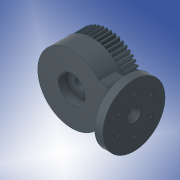
# Autodesk Inventor part: BA013
Saved by Autodesk Inventor 2017 SP1 (Build 210196100, 196)
## iProperties
Created: 2017-06-27
Part Number: BA013
Material: ABS Plastic
Document SubType Name: Modeling
Designer: zallen
Density: 1.06 g/cm^3
Appearance: CR Dark Blue
Author: zallen
Autodesk Inventor part; units mm, degrees
ref_plane "YZ Plane" through (0, 0, 0) normal (1, 0, 0) x (0, 1, 0)
ref_plane "XZ Plane" through (0, 0, 0) normal (0, 1, 0) x (-1, 0, 0)
ref_plane "XY Plane" through (0, 0, 0) normal (0, 0, 1) x (1, 0, 0)
sketch "Sketch1" plane through (0, 0, 0) normal (0, 0, 1) x (1, 0, 0)
  circle A0 centre (0, 0) radius 36.25
  circle A1 centre (0, 0) radius 7.5
  line L0 (0, 0) -> (67.2646, 0) construction
  arc A2 (40.2053, 0.75) -> (36.2053, 1.8) centre (34.4332, -13.095) ccw
  arc A3 (36.2053, -1.8) -> (40.2053, -0.75) centre (34.4332, 13.095) ccw
  arc A4 (40.2053, -0.75) -> (40.2053, 0.75) centre (20.2194, 0) ccw
  arc A5 (36.2053, -1.8) -> (36.2053, 1.8) centre (0, 0) ccw
  arc A6 (39.9823, 4.295) -> (39.7943, 5.7831) centre (20.0599, 2.5342) ccw
  arc A7 (39.7943, 5.7831) -> (35.6942, 6.3235) centre (35.8029, -8.6761) ccw
  arc A8 (36.1454, 2.7519) -> (39.9823, 4.295) centre (32.5204, 17.3073) ccw
  circle A9 centre (0, 0) radius 36.25
  arc A10 (39.1287, 9.2722) -> (38.7556, 10.7251) centre (19.5841, 5.0283) ccw
  arc A11 (38.7556, 10.7251) -> (34.6202, 10.7473) centre (36.608, -4.1204) ccw
  arc A12 (35.5155, 7.2604) -> (39.1287, 9.2722) centre (30.0948, 21.2467) ccw
  circle A13 centre (0, 0) radius 36.25
  arc A14 (37.658, 14.1032) -> (37.1058, 15.4979) centre (18.7995, 7.4432) ccw
  arc A15 (37.1058, 15.4979) -> (33.0002, 15.0017) centre (36.8357, 0.5003) ccw
  arc A16 (34.3254, 11.6545) -> (37.658, 14.1032) centre (27.1946, 24.8511) ccw
  circle A17 centre (0, 0) radius 36.25
  arc A18 (35.5935, 18.7118) -> (34.8708, 20.0263) centre (17.7184, 9.7407) ccw
  arc A19 (34.8708, 20.0263) -> (30.8598, 19.0194) centre (36.4826, 5.1131) ccw
  arc A20 (32.5941, 15.8647) -> (35.5935, 18.7118) centre (23.8655, 28.0635) ccw
  circle A21 centre (0, 0) radius 36.25
  arc A22 (32.9676, 23.0253) -> (32.0859, 24.2388) centre (16.3578, 11.8846) ccw
  arc A23 (32.0859, 24.2388) -> (28.2327, 22.7372) centre (35.554, 9.6453) ccw
  arc A24 (30.3487, 19.8247) -> (32.9676, 23.0253) centre (20.16, 30.8333) ccw
  circle A25 centre (0, 0) radius 36.25
  arc A26 (29.8218, 26.9757) -> (28.795, 28.0691) centre (14.7393, 13.8411) ccw
  arc A27 (28.795, 28.0691) -> (25.1603, 26.0964) centre (34.0648, 14.0253) ccw
  arc A28 (27.6247, 23.4721) -> (29.8218, 26.9757) centre (16.1366, 33.1169) ccw
  circle A29 centre (0, 0) radius 36.25
  arc A30 (26.2057, 30.5006) -> (25.0499, 31.4568) centre (12.8883, 15.5793) ccw
  arc A31 (25.0499, 31.4568) -> (21.6912, 29.044) centre (32.0384, 18.1842) ccw
  arc A32 (24.465, 26.7493) -> (26.2057, 30.5006) centre (11.8587, 34.8783) ccw
  circle A33 centre (0, 0) radius 36.25
  arc A34 (22.1763, 33.5446) -> (20.9098, 34.3483) centre (10.8341, 17.0718) ccw
  arc A35 (20.9098, 34.3483) -> (17.88, 31.5336) centre (29.5066, 22.0563) ccw
  arc A36 (20.9196, 29.6046) -> (22.1763, 33.5446) centre (7.3938, 36.0895) ccw
  circle A37 centre (0, 0) radius 36.25
  arc A38 (17.7972, 36.0595) -> (16.44, 36.6982) centre (8.609, 18.295) ccw
  arc A39 (16.44, 36.6982) -> (13.7868, 33.5259) centre (26.5096, 25.5805) ccw
  arc A40 (17.0441, 31.9931) -> (17.7972, 36.0595) centre (2.8123, 36.7316) ccw
  circle A41 centre (0, 0) radius 36.25
  arc A42 (13.1374, 38.0057) -> (11.7108, 38.4693) centre (6.2481, 19.2297) ccw
  arc A43 (11.7108, 38.4693) -> (9.4761, 34.9895) centre (23.0945, 28.7013) ccw
  arc A44 (12.8999, 33.877) -> (13.1374, 38.0057) centre (-1.8136, 36.7945) ccw
  circle A45 centre (0, 0) radius 36.25
  arc A46 (8.2704, 39.3526) -> (6.797, 39.6337) centre (3.7887, 19.8612) ccw
  arc A47 (6.797, 39.6337) -> (5.0161, 35.9013) centre (19.3151, 31.3695) ccw
  arc A48 (8.5523, 35.2267) -> (8.2704, 39.3526) centre (-6.4109, 36.277) ccw
  circle A49 centre (0, 0) radius 36.25
  arc A50 (3.273, 40.0789) -> (1.776, 40.173) centre (1.2696, 20.1795) ccw
  arc A51 (1.776, 40.173) -> (0.4769, 36.2469) centre (15.2312, 33.543) ccw
  arc A52 (4.0698, 36.0208) -> (3.273, 40.0789) centre (-10.907, 35.1875) ccw
  circle A53 centre (0, 0) radius 36.25
  arc A54 (-1.776, 40.173) -> (-3.273, 40.0789) centre (-1.2696, 20.1795) ccw
  arc A55 (-3.273, 40.0789) -> (-4.0698, 36.0208) centre (10.907, 35.1875) ccw
  arc A56 (-0.4769, 36.2469) -> (-1.776, 40.173) centre (-15.2312, 33.543) ccw
  circle A57 centre (0, 0) radius 36.25
  arc A58 (-6.797, 39.6337) -> (-8.2704, 39.3526) centre (-3.7887, 19.8612) ccw
  arc A59 (-8.2704, 39.3526) -> (-8.5523, 35.2267) centre (6.4109, 36.277) ccw
  arc A60 (-5.0161, 35.9013) -> (-6.797, 39.6337) centre (-19.3151, 31.3695) ccw
  circle A61 centre (0, 0) radius 36.25
  arc A62 (-11.7108, 38.4693) -> (-13.1374, 38.0057) centre (-6.2481, 19.2297) ccw
  arc A63 (-13.1374, 38.0057) -> (-12.8999, 33.877) centre (1.8136, 36.7945) ccw
  arc A64 (-9.4761, 34.9895) -> (-11.7108, 38.4693) centre (-23.0945, 28.7013) ccw
  circle A65 centre (0, 0) radius 36.25
  arc A66 (-16.44, 36.6982) -> (-17.7972, 36.0595) centre (-8.609, 18.295) ccw
  arc A67 (-17.7972, 36.0595) -> (-17.0441, 31.9931) centre (-2.8123, 36.7316) ccw
  arc A68 (-13.7868, 33.5259) -> (-16.44, 36.6982) centre (-26.5096, 25.5805) ccw
  circle A69 centre (0, 0) radius 36.25
  arc A70 (-20.9098, 34.3483) -> (-22.1763, 33.5446) centre (-10.8341, 17.0718) ccw
  arc A71 (-22.1763, 33.5446) -> (-20.9196, 29.6046) centre (-7.3938, 36.0895) ccw
  arc A72 (-17.88, 31.5336) -> (-20.9098, 34.3483) centre (-29.5066, 22.0563) ccw
  circle A73 centre (0, 0) radius 36.25
  arc A74 (-25.0499, 31.4568) -> (-26.2057, 30.5006) centre (-12.8883, 15.5793) ccw
  arc A75 (-26.2057, 30.5006) -> (-24.465, 26.7493) centre (-11.8587, 34.8783) ccw
  arc A76 (-21.6912, 29.044) -> (-25.0499, 31.4568) centre (-32.0384, 18.1842) ccw
  circle A77 centre (0, 0) radius 36.25
  arc A78 (-28.795, 28.0691) -> (-29.8218, 26.9757) centre (-14.7393, 13.8411) ccw
  arc A79 (-29.8218, 26.9757) -> (-27.6247, 23.4721) centre (-16.1366, 33.1169) ccw
  arc A80 (-25.1603, 26.0964) -> (-28.795, 28.0691) centre (-34.0648, 14.0253) ccw
  circle A81 centre (0, 0) radius 36.25
  arc A82 (-32.0859, 24.2388) -> (-32.9676, 23.0253) centre (-16.3578, 11.8846) ccw
  arc A83 (-32.9676, 23.0253) -> (-30.3487, 19.8247) centre (-20.16, 30.8333) ccw
  arc A84 (-28.2327, 22.7372) -> (-32.0859, 24.2388) centre (-35.554, 9.6453) ccw
  circle A85 centre (0, 0) radius 36.25
  arc A86 (-34.8708, 20.0263) -> (-35.5935, 18.7118) centre (-17.7184, 9.7407) ccw
  arc A87 (-35.5935, 18.7118) -> (-32.5941, 15.8647) centre (-23.8655, 28.0635) ccw
  arc A88 (-30.8598, 19.0194) -> (-34.8708, 20.0263) centre (-36.4826, 5.1131) ccw
  circle A89 centre (0, 0) radius 36.25
  arc A90 (-37.1058, 15.4979) -> (-37.658, 14.1032) centre (-18.7995, 7.4432) ccw
  arc A91 (-37.658, 14.1032) -> (-34.3254, 11.6545) centre (-27.1946, 24.8511) ccw
  arc A92 (-33.0002, 15.0017) -> (-37.1058, 15.4979) centre (-36.8357, 0.5003) ccw
  circle A93 centre (0, 0) radius 36.25
  arc A94 (-38.7556, 10.7251) -> (-39.1287, 9.2722) centre (-19.5841, 5.0283) ccw
  arc A95 (-39.1287, 9.2722) -> (-35.5155, 7.2604) centre (-30.0948, 21.2467) ccw
  arc A96 (-34.6202, 10.7473) -> (-38.7556, 10.7251) centre (-36.608, -4.1204) ccw
  circle A97 centre (0, 0) radius 36.25
  arc A98 (-39.7943, 5.7831) -> (-39.9823, 4.295) centre (-20.0599, 2.5342) ccw
  arc A99 (-39.9823, 4.295) -> (-36.1454, 2.7519) centre (-32.5204, 17.3073) ccw
  arc A100 (-35.6942, 6.3235) -> (-39.7943, 5.7831) centre (-35.8029, -8.6761) ccw
  circle A101 centre (0, 0) radius 36.25
  arc A102 (-40.2053, 0.75) -> (-40.2053, -0.75) centre (-20.2194, 0) ccw
  arc A103 (-40.2053, -0.75) -> (-36.2053, -1.8) centre (-34.4332, 13.095) ccw
  arc A104 (-36.2053, 1.8) -> (-40.2053, 0.75) centre (-34.4332, -13.095) ccw
  circle A105 centre (0, 0) radius 36.25
  arc A106 (-39.9823, -4.295) -> (-39.7943, -5.7831) centre (-20.0599, -2.5342) ccw
  arc A107 (-39.7943, -5.7831) -> (-35.6942, -6.3235) centre (-35.8029, 8.6761) ccw
  arc A108 (-36.1454, -2.7519) -> (-39.9823, -4.295) centre (-32.5204, -17.3073) ccw
  circle A109 centre (0, 0) radius 36.25
  arc A110 (-39.1287, -9.2722) -> (-38.7556, -10.7251) centre (-19.5841, -5.0283) ccw
  arc A111 (-38.7556, -10.7251) -> (-34.6202, -10.7473) centre (-36.608, 4.1204) ccw
  arc A112 (-35.5155, -7.2604) -> (-39.1287, -9.2722) centre (-30.0948, -21.2467) ccw
  circle A113 centre (0, 0) radius 36.25
  arc A114 (-37.658, -14.1032) -> (-37.1058, -15.4979) centre (-18.7995, -7.4432) ccw
  arc A115 (-37.1058, -15.4979) -> (-33.0002, -15.0017) centre (-36.8357, -0.5003) ccw
  arc A116 (-34.3254, -11.6545) -> (-37.658, -14.1032) centre (-27.1946, -24.8511) ccw
  circle A117 centre (0, 0) radius 36.25
  arc A118 (-35.5935, -18.7118) -> (-34.8708, -20.0263) centre (-17.7184, -9.7407) ccw
  arc A119 (-34.8708, -20.0263) -> (-30.8598, -19.0194) centre (-36.4826, -5.1131) ccw
  arc A120 (-32.5941, -15.8647) -> (-35.5935, -18.7118) centre (-23.8655, -28.0635) ccw
  circle A121 centre (0, 0) radius 36.25
  arc A122 (-32.9676, -23.0253) -> (-32.0859, -24.2388) centre (-16.3578, -11.8846) ccw
  arc A123 (-32.0859, -24.2388) -> (-28.2327, -22.7372) centre (-35.554, -9.6453) ccw
  arc A124 (-30.3487, -19.8247) -> (-32.9676, -23.0253) centre (-20.16, -30.8333) ccw
  circle A125 centre (0, 0) radius 36.25
  arc A126 (-29.8218, -26.9757) -> (-28.795, -28.0691) centre (-14.7393, -13.8411) ccw
  arc A127 (-28.795, -28.0691) -> (-25.1603, -26.0964) centre (-34.0648, -14.0253) ccw
  arc A128 (-27.6247, -23.4721) -> (-29.8218, -26.9757) centre (-16.1366, -33.1169) ccw
  circle A129 centre (0, 0) radius 36.25
  arc A130 (-26.2057, -30.5006) -> (-25.0499, -31.4568) centre (-12.8883, -15.5793) ccw
  arc A131 (-25.0499, -31.4568) -> (-21.6912, -29.044) centre (-32.0384, -18.1842) ccw
  arc A132 (-24.465, -26.7493) -> (-26.2057, -30.5006) centre (-11.8587, -34.8783) ccw
  circle A133 centre (0, 0) radius 36.25
  arc A134 (-22.1763, -33.5446) -> (-20.9098, -34.3483) centre (-10.8341, -17.0718) ccw
  arc A135 (-20.9098, -34.3483) -> (-17.88, -31.5336) centre (-29.5066, -22.0563) ccw
  arc A136 (-20.9196, -29.6046) -> (-22.1763, -33.5446) centre (-7.3938, -36.0895) ccw
  circle A137 centre (0, 0) radius 36.25
  arc A138 (-17.7972, -36.0595) -> (-16.44, -36.6982) centre (-8.609, -18.295) ccw
  arc A139 (-16.44, -36.6982) -> (-13.7868, -33.5259) centre (-26.5096, -25.5805) ccw
  arc A140 (-17.0441, -31.9931) -> (-17.7972, -36.0595) centre (-2.8123, -36.7316) ccw
  circle A141 centre (0, 0) radius 36.25
  arc A142 (-13.1374, -38.0057) -> (-11.7108, -38.4693) centre (-6.2481, -19.2297) ccw
  arc A143 (-11.7108, -38.4693) -> (-9.4761, -34.9895) centre (-23.0945, -28.7013) ccw
  arc A144 (-12.8999, -33.877) -> (-13.1374, -38.0057) centre (1.8136, -36.7945) ccw
  circle A145 centre (0, 0) radius 36.25
  arc A146 (-8.2704, -39.3526) -> (-6.797, -39.6337) centre (-3.7887, -19.8612) ccw
  arc A147 (-6.797, -39.6337) -> (-5.0161, -35.9013) centre (-19.3151, -31.3695) ccw
  arc A148 (-8.5523, -35.2267) -> (-8.2704, -39.3526) centre (6.4109, -36.277) ccw
  circle A149 centre (0, 0) radius 36.25
  arc A150 (-3.273, -40.0789) -> (-1.776, -40.173) centre (-1.2696, -20.1795) ccw
  arc A151 (-1.776, -40.173) -> (-0.4769, -36.2469) centre (-15.2312, -33.543) ccw
  arc A152 (-4.0698, -36.0208) -> (-3.273, -40.0789) centre (10.907, -35.1875) ccw
  circle A153 centre (0, 0) radius 36.25
  arc A154 (1.776, -40.173) -> (3.273, -40.0789) centre (1.2696, -20.1795) ccw
  arc A155 (3.273, -40.0789) -> (4.0698, -36.0208) centre (-10.907, -35.1875) ccw
  arc A156 (0.4769, -36.2469) -> (1.776, -40.173) centre (15.2312, -33.543) ccw
  circle A157 centre (0, 0) radius 36.25
  arc A158 (6.797, -39.6337) -> (8.2704, -39.3526) centre (3.7887, -19.8612) ccw
  arc A159 (8.2704, -39.3526) -> (8.5523, -35.2267) centre (-6.4109, -36.277) ccw
  arc A160 (5.0161, -35.9013) -> (6.797, -39.6337) centre (19.3151, -31.3695) ccw
  circle A161 centre (0, 0) radius 36.25
  arc A162 (11.7108, -38.4693) -> (13.1374, -38.0057) centre (6.2481, -19.2297) ccw
  arc A163 (13.1374, -38.0057) -> (12.8999, -33.877) centre (-1.8136, -36.7945) ccw
  arc A164 (9.4761, -34.9895) -> (11.7108, -38.4693) centre (23.0945, -28.7013) ccw
  circle A165 centre (0, 0) radius 36.25
  arc A166 (16.44, -36.6982) -> (17.7972, -36.0595) centre (8.609, -18.295) ccw
  arc A167 (17.7972, -36.0595) -> (17.0441, -31.9931) centre (2.8123, -36.7316) ccw
  arc A168 (13.7868, -33.5259) -> (16.44, -36.6982) centre (26.5096, -25.5805) ccw
  circle A169 centre (0, 0) radius 36.25
  arc A170 (20.9098, -34.3483) -> (22.1763, -33.5446) centre (10.8341, -17.0718) ccw
  arc A171 (22.1763, -33.5446) -> (20.9196, -29.6046) centre (7.3938, -36.0895) ccw
  arc A172 (17.88, -31.5336) -> (20.9098, -34.3483) centre (29.5066, -22.0563) ccw
  circle A173 centre (0, 0) radius 36.25
  arc A174 (25.0499, -31.4568) -> (26.2057, -30.5006) centre (12.8883, -15.5793) ccw
  arc A175 (26.2057, -30.5006) -> (24.465, -26.7493) centre (11.8587, -34.8783) ccw
  arc A176 (21.6912, -29.044) -> (25.0499, -31.4568) centre (32.0384, -18.1842) ccw
  circle A177 centre (0, 0) radius 36.25
  arc A178 (28.795, -28.0691) -> (29.8218, -26.9757) centre (14.7393, -13.8411) ccw
  arc A179 (29.8218, -26.9757) -> (27.6247, -23.4721) centre (16.1366, -33.1169) ccw
  arc A180 (25.1603, -26.0964) -> (28.795, -28.0691) centre (34.0648, -14.0253) ccw
  circle A181 centre (0, 0) radius 36.25
  arc A182 (32.0859, -24.2388) -> (32.9676, -23.0253) centre (16.3578, -11.8846) ccw
  arc A183 (32.9676, -23.0253) -> (30.3487, -19.8247) centre (20.16, -30.8333) ccw
  arc A184 (28.2327, -22.7372) -> (32.0859, -24.2388) centre (35.554, -9.6453) ccw
  circle A185 centre (0, 0) radius 36.25
  arc A186 (34.8708, -20.0263) -> (35.5935, -18.7118) centre (17.7184, -9.7407) ccw
  arc A187 (35.5935, -18.7118) -> (32.5941, -15.8647) centre (23.8655, -28.0635) ccw
  arc A188 (30.8598, -19.0194) -> (34.8708, -20.0263) centre (36.4826, -5.1131) ccw
  circle A189 centre (0, 0) radius 36.25
  arc A190 (37.1058, -15.4979) -> (37.658, -14.1032) centre (18.7995, -7.4432) ccw
  arc A191 (37.658, -14.1032) -> (34.3254, -11.6545) centre (27.1946, -24.8511) ccw
  arc A192 (33.0002, -15.0017) -> (37.1058, -15.4979) centre (36.8357, -0.5003) ccw
  circle A193 centre (0, 0) radius 36.25
  arc A194 (38.7556, -10.7251) -> (39.1287, -9.2722) centre (19.5841, -5.0283) ccw
  arc A195 (39.1287, -9.2722) -> (35.5155, -7.2604) centre (30.0948, -21.2467) ccw
  arc A196 (34.6202, -10.7473) -> (38.7556, -10.7251) centre (36.608, 4.1204) ccw
  circle A197 centre (0, 0) radius 36.25
  arc A198 (39.7943, -5.7831) -> (39.9823, -4.295) centre (20.0599, -2.5342) ccw
  arc A199 (39.9823, -4.295) -> (36.1454, -2.7519) centre (32.5204, -17.3073) ccw
  arc A200 (35.6942, -6.3235) -> (39.7943, -5.7831) centre (35.8029, 8.6761) ccw
  circle A201 centre (0, 0) radius 36.25
  point P0 (40.2194, 0)
  point P1 (39.9022, 5.0408)
  point P2 (38.9558, 10.0021)
  point P3 (37.395, 14.8057)
  point P4 (35.2445, 19.3758)
  point P5 (32.5381, 23.6403)
  point P6 (29.3186, 27.532)
  point P7 (25.6368, 30.9895)
  point P8 (21.5506, 33.9583)
  point P9 (17.1246, 36.3916)
  point P10 (12.4285, 38.2509)
  point P11 (7.5364, 39.507)
  point P12 (2.5254, 40.14)
  point P13 (-2.5254, 40.14)
  point P14 (-7.5364, 39.507)
  point P15 (-12.4285, 38.2509)
  point P16 (-17.1246, 36.3916)
  point P17 (-21.5506, 33.9583)
  point P18 (-25.6368, 30.9895)
  point P19 (-29.3186, 27.532)
  point P20 (-32.5381, 23.6403)
  point P21 (-35.2445, 19.3758)
  point P22 (-37.395, 14.8057)
  point P23 (-38.9558, 10.0021)
  point P24 (-39.9022, 5.0408)
  point P25 (-40.2194, 0)
  point P26 (-39.9022, -5.0408)
  point P27 (-38.9558, -10.0021)
  point P28 (-37.395, -14.8057)
  point P29 (-35.2445, -19.3758)
  point P30 (-32.5381, -23.6403)
  point P31 (-29.3186, -27.532)
  point P32 (-25.6368, -30.9895)
  point P33 (-21.5506, -33.9583)
  point P34 (-17.1246, -36.3916)
  point P35 (-12.4285, -38.2509)
  point P36 (-7.5364, -39.507)
  point P37 (-2.5254, -40.14)
  point P38 (2.5254, -40.14)
  point P39 (7.5364, -39.507)
  point P40 (12.4285, -38.2509)
  point P41 (17.1246, -36.3916)
  point P42 (21.5506, -33.9583)
  point P43 (25.6368, -30.9895)
  point P44 (29.3186, -27.532)
  point P45 (32.5381, -23.6403)
  point P46 (35.2445, -19.3758)
  point P47 (37.395, -14.8057)
  point P48 (38.9558, -10.0021)
  point P49 (39.9022, -5.0408)
  dimension "d0" = 72.5
  dimension "d1" = 15
  dimension "d2" = 15
  dimension "d3" = 15
  dimension "d4" = 20
  dimension "d5" = 4
  dimension "d10" = 1.8
  dimension "d12" = 1.5
  dimension "d15" = 360
  constraints: 403 point on circle, 202 centre point, 2 coincident, 2 end point, 2 vertical alignment, 1 concentric, 1 horizontal, 1 point on line, 651 other
  measures "d0" diameter of A0
  measures "d1" diameter of A1
  measures "d2" radius of A2
  measures "d3" radius of A3
  measures "d4" radius of A4
  measures "d5" horizontal distance of A2.start A0.start
  measures "d10" distance from line of L0 A0.start
  measures "d12" distance of A3.end A2.start
extrude "Extrusion1" add sketch "Sketch1" along normal blind 20
sketch "Sketch2" plane through (0, 0, 20) normal (0, 0, 1) x (1, 0, 0)
  circle A0 centre (0, 0) radius 7.5 projected
  circle A1 centre (0, 0) radius 41
  dimension "d19" = 82
  constraints: 1 centre point, 1 coincident
  measures "d19" diameter of A1
extrude "Extrusion2" add sketch "Sketch2" along normal blind 15
sketch "Sketch11" plane through (0, 0, 35) normal (0, 0, 1) x (1, 0, 0)
  circle A0 centre (0, 0) radius 7.5 projected
  circle A1 centre (0, 0) radius 41
  dimension "d59" = 82
  constraints: 1 centre point, 1 coincident
  measures "d59" diameter of A1
extrude "Extrusion11" add sketch "Sketch11" along normal blind 10
sketch "Sketch12" plane through (0, 0, 45) normal (0, 0, 1) x (1, 0, 0)
  circle A0 centre (0, 0) radius 16.25
  dimension "d62" = 32.5
  constraints: 1 centre point, 1 coincident
  measures "d62" diameter of A0
extrude "Extrusion12" cut sketch "Sketch12" against normal blind 11
sketch "Sketch13" plane through (0, 0, 0) normal (0, 0, -1) x (-1, 0, 0)
  circle A0 centre (0, 0) radius 16.25 projected
extrude "Extrusion13" cut sketch "Sketch13" against normal blind 11
sketch "Sketch14" plane through (0, 0, 45) normal (0, 0, 1) x (1, 0, 0)
  line L0 (0, -25) -> (55, -25)
  line L1 (55, -25) -> (55, 25)
  line L2 (55, 25) -> (0, 25)
  line L3 (0, 25) -> (0, -25)
  circle A0 centre (0, 0) radius 16.25 projected
  circle A1 centre (0, 0) radius 16.25 projected
  arc A2 (0, -16.25) -> (0, 16.25) centre (0, 0) ccw
  dimension "d67" = 55
  dimension "d68" = 50
  constraints: 8 end point, 6 point on circle, 2 midpoint, 2 parallel, 2 point on line, 1 centre point, 1 concentric, 1 horizontal, 1 perpendicular
  measures "d67" distance of L2.end L1.end
  measures "d68" distance of L1.end L0.end
extrude "Extrusion15" add sketch "Sketch14" against normal blind 20 contours L3 A0 L2 L1 L0
sketch "Sketch15" plane through (55, -25, 45) normal (1, 0, 0) x (0, 0, -1)
  circle A0 centre (10, 25) radius 37.5
  line L0 (0, 0) -> (20, 0) construction
  line L1 (20, 50) -> (20, 0) construction
  point P0 (10, 0)
  point P1 (20, 25)
  dimension "d93" = 75
  constraints: 2 midpoint, 1 centre point, 1 horizontal alignment, 1 vertical alignment
  measures "d93" diameter of A0
extrude "Extrusion16" add sketch "Sketch15" along normal blind 10
sketch "Sketch16" plane through (65, -25, 45) normal (1, 0, 0) x (0, 0, -1)
  circle A0 centre (10, 25) radius 37.5 construction
  line L0 (10, 25) -> (10, 2.5) construction
  circle A1 centre (10, 2.5) radius 2.5
  line L1 (10, 25) -> (29.4856, 13.75) construction
  circle A2 centre (29.4856, 13.75) radius 2.5
  line L2 (10, 25) -> (29.4856, 36.25) construction
  circle A3 centre (29.4856, 36.25) radius 2.5
  line L3 (10, 25) -> (10, 47.5) construction
  circle A4 centre (10, 47.5) radius 2.5
  line L4 (10, 25) -> (-9.4856, 36.25) construction
  circle A5 centre (-9.4856, 36.25) radius 2.5
  line L5 (10, 25) -> (-9.4856, 13.75) construction
  circle A6 centre (-9.4856, 13.75) radius 2.5
  dimension "d96" = 22.5
  dimension "d97" = 5
  dimension "d100" = 360
  constraints: 12 end point, 8 coincident, 6 centre point, 1 vertical, 29 other
  measures "d96" distance of L0.start L0.end
  measures "d97" diameter of A1
extrude "Extrusion17" cut sketch "Sketch16" against normal blind 10
sketch "Sketch18" plane through (65, 0, 35) normal (1, 0, 0) x (0, 0, -1)
  circle A0 centre (0, 0) radius 37.5 construction
  circle A1 centre (0, 0) radius 7.5
  dimension "d102" = 15
  constraints: 1 centre point, 1 coincident
  measures "d102" diameter of A1
extrude "Extrusion19" cut sketch "Sketch18" against normal blind 10
body "Solid1"
